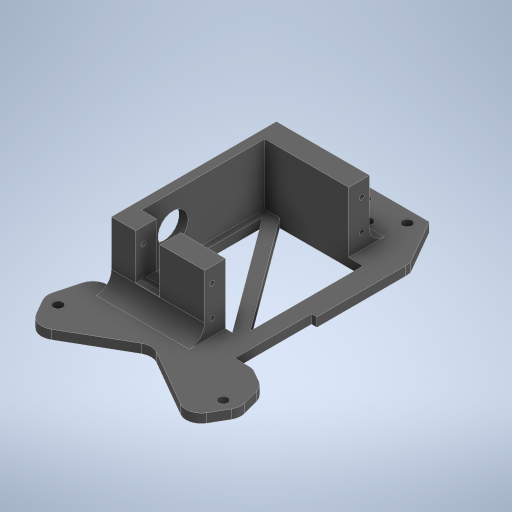
# Autodesk Inventor part: upper_arm_base
Saved by Autodesk Inventor 2024.1 (Build 281209000, 209)
## iProperties
Created: 2025-03-03
Part Number: upper_arm_base
Material: 一般
Document SubType Name: Modeling
Designer: hibik
Density: 1 g/cm^3
Appearance: 既定
Author: hibik
Autodesk Inventor part; units mm, degrees
ref_plane "XZ Plane" through (0, 0, 0) normal (0, 1, 0) x (-1, 0, 0)
ref_plane "XY Plane" through (0, 0, 0) normal (0, 0, 1) x (1, 0, 0)
ref_plane "作業平面1" through (7.8, 0, 0) normal (1, 0, 0) x (0, 1, 0)
sketch "スケッチ1" plane through (7.8, 0, 0) normal (1, 0, 0) x (0, 1, 0)
  line L0 (0, 27.3) -> (-20.1, 27.3)
  line L1 (-20.1, 27.3) -> (-20.1, 20.4)
  line L2 (-20.1, 20.4) -> (0, 20.4)
  line L3 (0, 20.4) -> (0, 27.3)
  line L4 (0, -20.4) -> (-20.1, -20.4)
  line L5 (-20.1, -20.4) -> (-20.1, -27.3)
  line L6 (-20.1, -27.3) -> (0, -27.3)
  line L7 (0, -27.3) -> (0, -20.4)
  line L8 (0, -38.22) -> (0, 38.22) projected
  line L9 (-24.12, 0) -> (4.02, 0) projected
  point P0 (0, 0)
  dimension "d1" = 40.8
  dimension "d3" = 20.1
  dimension "d13" = 6.9
  constraints: 16 end point, 4 parallel, 3 collinear, 2 horizontal, 2 perpendicular, 1 point on line, 1 other
  measures "d1" distance between parallel lines of L4 L2
  measures "d3" distance of L5.end L6.end
  measures "d13" distance of L2.end L0.start
extrude "押し出し1" add sketch "スケッチ1" against normal blind 27.8
sketch "スケッチ2" plane through (-20, 0, 0) normal (-1, 0, 0) x (0, 0, 1)
  line L0 (27.3, 0) -> (27.3, -20.1) projected
  line L1 (-27.3, -20.1) -> (-20.4, -20.1) projected
  line L2 (27.3, 0) -> (-27.3, 0)
  line L3 (-27.3, 0) -> (-27.3, -20.1)
  line L4 (-27.3, -20.1) -> (27.3, -20.1)
  line L5 (27.3, -20.1) -> (27.3, 0)
  point P0 (0, 0)
  constraints: 8 end point, 2 parallel, 1 horizontal, 1 perpendicular
extrude "押し出し2" add sketch "スケッチ2" along normal blind 3
sketch "スケッチ3" plane through (-23, 0, 0) normal (-1, 0, 0) x (0, 0, 1)
  circle A0 centre (9.9, -10.5) radius 5
  line L0 (27.3, 0) -> (-27.3, 0) projected
  line L1 (20.4, 0) -> (20.4, -20.1) projected
  point P0 (0, 0)
  dimension "d8" = 10
  dimension "d9" = 10.5
  dimension "d10" = 10.5
  constraints: 1 centre point
  measures "d8" diameter of A0
  measures "d9" distance from line of L0 A0.centre
  measures "d10" distance from line of L1 A0.centre
extrude "押し出し3" cut sketch "スケッチ3" against normal through all
sketch "スケッチ7" plane through (7.8, 0, 0) normal (1, 0, 0) x (0, 0, -1)
  arc A0 (-26.6208, -6.3) -> (-26.6208, -3.8) centre (-24.75, -5.05) ccw projected
  arc A1 (-26.6208, -16.3) -> (-26.6208, -13.8) centre (-24.75, -15.05) ccw projected
  arc A2 (26.6208, -3.8) -> (26.6208, -6.3) centre (24.75, -5.05) ccw projected
  arc A3 (26.6208, -13.8) -> (26.6208, -16.3) centre (24.75, -15.05) ccw projected
  circle A4 centre (-24.75, -5.05) radius 0.85
  circle A5 centre (-24.75, -15.05) radius 0.85
  circle A6 centre (24.75, -5.05) radius 0.85
  circle A7 centre (24.75, -15.05) radius 0.85
  point P0 (0, 0)
  dimension "d25" = 1.7
  constraints: 4 centre point, 3 coincident, 3 equal radius, 1 concentric
  measures "d25" diameter of A4
extrude "押し出し6" cut sketch "スケッチ7" against normal through all
sketch "スケッチ9" plane through (7.8, -20.1, -27.3) normal (0, -1, 0) x (1, 0, 0)
  line L0 (-32.5673, -16.6603) -> (18.1673, -16.6603)
  line L1 (18.1673, -16.6603) -> (55.6673, 48.2917)
  line L2 (55.6673, 48.2917) -> (30.3, 92.2291)
  line L3 (30.3, 92.2291) -> (-44.7, 92.2291)
  line L4 (-44.7, 92.2291) -> (-70.0673, 48.2917)
  line L5 (-70.0673, 48.2917) -> (-32.5673, -16.6603)
  line L6 (0, 0) -> (-30.8, 0) projected
  line L7 (11.8, 54.6) -> (-26.2, 54.6)
  line L8 (-26.2, 54.6) -> (-26.2, 0) construction
  line L9 (-26.2, 0) -> (11.8, 0)
  line L10 (11.8, 0) -> (11.8, 54.6)
  line L11 (0, 6.9) -> (0, 0) projected
  line L12 (0, 54.6) -> (-30.8, 54.6) projected
  line L13 (-142.2, 119.2291) -> (-7.2, -114.5977)
  line L14 (-7.2, -114.5977) -> (127.8, 119.2291)
  line L15 (-37.5673, -8) -> (-27.175, -2)
  line L16 (-27.175, -2) -> (-7.2, -2)
  line L17 (-142.2, 119.2291) -> (127.8, 119.2291)
  line L18 (-7.2, -2) -> (-7.2, -16.6603) construction
  line L19 (23.1673, -8) -> (12.775, -2)
  line L20 (12.775, -2) -> (-7.2, -2)
  line L21 (-26.0203, -2) -> (-17.5562, -16.6603)
  line L22 (11.6203, -2) -> (3.1562, -16.6603)
  line L23 (-57.3837, 70.2604) -> (36.9173, 15.8157) construction
  line L24 (42.9837, 70.2604) -> (-51.3173, 15.8157) construction
  line L25 (50.6673, 39.6314) -> (40.275, 45.6314)
  line L26 (40.275, 45.6314) -> (30.2875, 62.9303)
  line L27 (20.3, 80.2291) -> (30.2875, 62.9303)
  line L28 (20.3, 92.2291) -> (20.3, 80.2291)
  line L29 (20.8774, 79.2291) -> (37.8056, 79.2291)
  line L30 (39.6977, 46.6314) -> (48.1618, 61.2917)
  line L31 (-34.7, 92.2291) -> (-34.7, 80.2291)
  line L32 (-34.7, 80.2291) -> (-44.6875, 62.9303)
  line L33 (-54.675, 45.6314) -> (-44.6875, 62.9303)
  line L34 (-65.0673, 39.6314) -> (-54.675, 45.6314)
  line L35 (-54.0977, 46.6314) -> (-62.5618, 61.2917)
  line L36 (-35.2774, 79.2291) -> (-52.2056, 79.2291)
  line L37 (-54.0977, 46.6314) -> (-26.0203, -2) construction
  line L38 (11.6203, -2) -> (39.6977, 46.6314) construction
  line L39 (-35.2774, 79.2291) -> (20.8774, 79.2291) construction
  line L40 (18.5679, 79.2291) -> (38.543, 44.6314)
  line L41 (-32.9679, 79.2291) -> (-52.943, 44.6314)
  line L42 (-34.7, 80.2291) -> (-7.2, 64.352)
  line L43 (-7.2, 64.352) -> (20.3, 80.2291)
  line L44 (11.8, 29.1913) -> (40.275, 45.6314)
  line L45 (-54.675, 45.6314) -> (-30.8, 31.8472)
  line L46 (-30.8, 0) -> (-30.8, 54.6) projected
  line L47 (-26.0203, -2) -> (-27.175, 0)
  line L48 (11.6203, -2) -> (11.8, 0)
  point P0 (-7.8, 27.3)
  point P1 (-7.2, 92.2291)
  point P2 (-7.2, 0)
  point P3 (-7.2, 41.2868)
  point P4 (-32.9679, 79.2291)
  point P5 (-52.943, 44.6314)
  dimension "d29" = 38
  dimension "d30" = 26.2
  dimension "d34" = 270
  dimension "d35" = 75
  dimension "d37" = 27
  dimension "d38" = 27
  dimension "d40" = 10
  dimension "d41" = 12
  dimension "d42" = 27
  dimension "d43" = 1
  dimension "d44" = 1
  dimension "d45" = 2
  dimension "d48" = 360
  dimension "d50" = 2
  dimension "d51" = 2
  constraints: 90 end point, 17 point on line, 9 parallel, 7 midpoint, 7 perpendicular, 6 horizontal, 5 equal length, 2 symmetric about line, 1 coincident, 1 collinear, 1 vertical alignment, 46 other
  measures "d29" distance of L8.end L9.end
  measures "d30" distance between parallel lines of L8 L11
  measures "d34" distance of L14.end L13.start
  measures "d35" distance of L2.end L3.end
  measures "d37" distance between parallel lines of L13 L5
  measures "d38" distance between parallel lines of L14 L1
  measures "d40" distance from line of L0.start L15
  measures "d41" distance from line of L15.end L5
  measures "d42" distance between parallel lines of L17 L3
  measures "d43" distance from line of L15.end L21
  measures "d44" distance from line of L20.start L22
  measures "d45" distance between parallel lines of L6 L16
  measures "d50" distance between parallel lines of L27 L40
  measures "d51" distance between parallel lines of L32 L41
extrude "押し出し7" add sketch "スケッチ9" along normal blind 3 contours L21 L16 L20 L22 L0 | L47 L6 L9 L48 L20 L16 | L6 L46 L12 L7 L10 L9 | L41 L42 L43 L40 L44 L10 L7 L12 L46 L45
sketch "スケッチ12" plane through (7.8, -20.1, -27.3) normal (0, 1, 0) x (1, 0, 0)
  line L0 (0, -47.7) -> (0, -54.6) projected
  line L1 (0, -54.6) -> (10, -54.6)
  line L2 (10, -54.6) -> (10, -29.6)
  line L3 (10, -29.6) -> (0, -29.6)
  line L4 (0, -29.6) -> (0, -54.6)
  line L5 (11.8, 0) -> (11.8, -29.1913) projected
  line L6 (10, -54.6) -> (16, -54.6)
  line L7 (16, -54.6) -> (16, -29.1913)
  line L8 (16, -29.1913) -> (10, -29.1913)
  line L9 (10, -29.1913) -> (10, -54.6)
  line L10 (0, -54.6) -> (-30.8, -54.6) projected
  line L11 (-30.8, -54.6) -> (-47.1876, -54.6)
  line L12 (-32.9679, -79.2291) -> (-52.943, -44.6314) projected
  line L13 (-52.943, -44.6314) -> (-30.8, -31.8472) projected
  line L14 (-30.8, -54.6) -> (-30.8, 0) projected
  point P0 (-7.8, -27.3)
  dimension "d59" = 25
  dimension "d60" = 10
  dimension "d61" = 6
  constraints: 18 end point, 4 parallel, 3 horizontal, 2 perpendicular, 2 point on line
  measures "d59" distance of L1.end L2.end
  measures "d60" distance of L0.end L1.end
  measures "d61" distance of L1.end L6.end
extrude "押し出し9" cut sketch "スケッチ12" against normal through all contours L2 L9 L8 L7 L6 | L11 L12 L13 L14
sketch "スケッチ13" plane through (7.8, -20.1, -27.3) normal (0, 1, 0) x (1, 0, 0)
  circle A0 centre (-0.2, 12.6603) radius 1.6
  circle A1 centre (-14.2, 12.6603) radius 1.6
  line L0 (-17.5562, 16.6603) -> (3.1562, 16.6603) projected
  line L1 (-7.2, 16.6603) -> (-7.2, 5.6822)
  line L2 (-17.5562, 16.6603) -> (3.1562, 16.6603) projected
  circle A2 centre (-34.5038, -68.5689) radius 1.6
  circle A3 centre (-44.4789, -51.2917) radius 1.6
  line L3 (-32.9679, -79.2291) -> (-52.943, -44.6314) projected
  line L4 (-42.9555, -61.9303) -> (-35.2404, -57.476)
  line L5 (-7.2, -64.352) -> (-32.9679, -79.2291) projected
  line L6 (-7.2, -64.352) -> (-7.2, -38.8829)
  circle A4 centre (20.1038, -68.5689) radius 1.6
  circle A5 centre (30.0789, -51.2917) radius 1.6
  point P0 (-7.8, -27.3)
  dimension "d64" = 3.2
  dimension "d65" = 4
  dimension "d66" = 7
  dimension "d75" = 10
  dimension "d76" = 4
  constraints: 6 centre point, 6 end point, 4 symmetric about line, 3 equal radius, 2 midpoint, 2 perpendicular, 1 vertical, 2 other
  measures "d64" diameter of A0
  measures "d65" distance from line of L0 A0.centre
  measures "d66" distance from line of L1 A0.centre
  measures "d75" distance from line of L5 A2.centre
  measures "d76" distance from line of L3 A2.centre
extrude "押し出し10" cut sketch "スケッチ13" against normal through all
sketch "スケッチ14" plane through (7.8, -20.1, -27.3) normal (0, 1, 0) x (1, 0, 0)
  line L0 (4.8, -47.7) -> (-25.8, -47.7)
  line L1 (-25.8, -47.7) -> (-25.8, -6.9)
  line L2 (-25.8, -6.9) -> (4.8, -6.9)
  line L3 (4.8, -6.9) -> (4.8, -47.7)
  line L4 (0, -47.7) -> (-27.8, -47.7) projected
  line L5 (-27.8, -47.7) -> (-27.8, -6.9) projected
  line L6 (0, -6.9) -> (-27.8, -6.9) projected
  line L7 (-30.8, -31.8472) -> (-30.8, 0) projected
  line L8 (11.8, 0) -> (11.8, -29.1913) projected
  line L9 (3.1906, -48.8873) -> (6.4094, -46.5127)
  line L10 (6.4094, -46.5127) -> (-23.6906, -5.7127)
  line L11 (-23.6906, -5.7127) -> (-26.9094, -8.0873)
  line L12 (-26.9094, -8.0873) -> (3.1906, -48.8873)
  line L13 (16, -54.6) -> (10, -54.6) projected
  line L14 (16, -54.6) -> (28.5907, -61.8692)
  line L15 (38.543, -44.6314) -> (18.5679, -79.2291) projected
  circle A0 centre (-14.2, 12.6603) radius 1.6 projected
  circle A1 centre (-0.2, 12.6603) radius 1.6 projected
  line L16 (16, -31.6162) -> (16, -54.6) projected
  line L17 (16, -54.6) -> (10, -54.6) projected
  line L18 (10, -54.6) -> (10, -29.1913) projected
  line L19 (10, -29.1913) -> (11.8, -29.1913) projected
  line L20 (11.8, 0) -> (11.8, -29.1913) projected
  line L21 (11.6203, 2) -> (11.8, 0) projected
  line L22 (3.1562, 16.6603) -> (11.6203, 2) projected
  line L23 (-17.5562, 16.6603) -> (3.1562, 16.6603) projected
  line L24 (-27.175, 0) -> (-17.5562, 16.6603) projected
  line L25 (0, 0) -> (-27.175, 0) projected
  line L26 (0, -6.9) -> (0, 0) projected
  line L27 (0, -6.9) -> (-27.8, -6.9) projected
  line L28 (-27.8, -6.9) -> (-27.8, -47.7) projected
  line L29 (0, -47.7) -> (-27.8, -47.7) projected
  line L30 (0, -54.6) -> (0, -47.7) projected
  line L31 (0, -54.6) -> (-30.8, -54.6) projected
  line L32 (-32.9679, -79.2291) -> (-47.1876, -54.6) projected
  line L33 (-7.2, -64.352) -> (-32.9679, -79.2291) projected
  line L34 (18.5679, -79.2291) -> (-7.2, -64.352) projected
  line L35 (38.543, -44.6314) -> (18.5679, -79.2291) projected
  line L36 (16, -31.6162) -> (38.543, -44.6314) projected
  circle A2 centre (-31.6735, -71.7906) radius 2.8438
  circle A3 centre (-40.8912, -49.9054) radius 3.5315
  line L37 (-30.8, -54.6) -> (-47.1876, -54.6) projected
  point P0 (-7.8, -27.3)
  point P1 (-22.8, -6.9)
  point P2 (-25.3, -6.9)
  point P3 (-22.8146, -6.9)
  point P4 (4.8, -44.3311)
  point P5 (2.3146, -47.7)
  point P6 (-25.8, -9.5911)
  dimension "d69" = 5
  dimension "d70" = 7
  dimension "d71" = 4
  constraints: 18 end point, 4 parallel, 3 perpendicular, 2 centre point, 2 collinear, 2 midpoint, 2 point on line, 1 horizontal
  measures "d69" distance between parallel lines of L7 L1
  measures "d70" distance between parallel lines of L8 L3
  measures "d71" distance between parallel lines of L12 L10
extrude "押し出し11" cut sketch "スケッチ14" against normal through all contours L0 L1 L12 | L10 L2 L3 | L14 L16 L36 L15
fillet "フィレット2" radius 5 2 edges at (-7.6, -20.1, 27.3) (-5.7875, -20.1, -27.3)
sketch "スケッチ16" plane through (7.8, -20.1, -27.3) normal (0, 1, 0) x (1, 0, 0)
  line L0 (-39.4555, -67.9924) -> (-36.8933, -58.4303)
  line L1 (-36.8933, -58.4303) -> (-46.4555, -55.8681)
  line L2 (-32.9679, -79.2291) -> (-52.943, -44.6314) projected
  line L3 (28.5907, -61.8692) -> (18.5679, -79.2291) projected
  line L4 (25.0907, -67.9314) -> (22.5285, -58.3692)
  line L5 (28.5907, -61.8692) -> (16, -54.6) projected
  line L6 (-36.8933, -58.4303) -> (-42.9555, -61.9303)
  line L7 (-36.8933, -58.4303) -> (-35.867, -54.6)
  line L8 (-35.867, -54.6) -> (-47.1876, -54.6)
  line L9 (-46.4555, -55.8681) -> (-47.1876, -54.6)
  line L10 (-30.8, -54.6) -> (-47.1876, -54.6) projected
  point P0 (-7.8, -27.3)
  dimension "d78" = 7
  dimension "d79" = 7
  dimension "d80" = 7
  dimension "d81" = 7
  constraints: 14 end point, 4 point on line, 2 equal length, 2 perpendicular, 1 collinear, 1 horizontal, 1 midpoint
  measures "d78" distance from line of L0.start L6
  measures "d79" distance from line of L0.end L2
  measures "d80" distance from line of L4.end L3
  measures "d81" distance from line of L4.start L5
extrude "押し出し12" cut sketch "スケッチ16" against normal through all
sketch "スケッチ17" plane through (-23, 0, 27.3) normal (0, 0, 1) x (1, 0, 0)
  line L0 (30.8, 0) -> (0, 0) projected
  line L1 (8, 0) -> (16, 0)
  line L2 (16, 0) -> (16, -15)
  line L3 (16, -15) -> (8, -15)
  line L4 (8, -15) -> (8, 0)
  line L5 (3, -5.5) -> (3, -15.5) projected
  line L6 (3, -20.1) -> (3, 0) projected
  line L7 (3, 0) -> (3, -20.1) projected
  point P0 (23, 0)
  dimension "d84" = 15
  dimension "d89" = 5
  dimension "d90" = 13
  constraints: 8 end point, 2 parallel, 1 horizontal, 1 perpendicular, 1 point on line
  measures "d84" distance of L1.end L2.end
  measures "d89" distance between parallel lines of L4 L6
  measures "d90" distance between parallel lines of L6 L2
extrude "押し出し13" cut sketch "スケッチ17" against normal up to surface (6.9 mm away)
sketch "スケッチ18" plane through (7.8, -20.1, -27.3) normal (0, 1, 0) x (1, 0, 0)
  circle A0 centre (-7.2, 6.6603) radius 1.6
  circle A1 centre (-0.2, 12.6603) radius 1.6 projected
  circle A2 centre (-14.2, 12.6603) radius 1.6 projected
  point P0 (-7.8, -27.3)
  dimension "d91" = 3.2
  dimension "d92" = 7
  dimension "d93" = 7
  dimension "d94" = 6
  constraints: 1 centre point
  measures "d91" diameter of A0
  measures "d92" horizontal distance of A0.centre A1.centre
  measures "d93" horizontal distance of A2.centre A0.centre
  measures "d94" vertical distance of A2.centre A0.centre
extrude "押し出し14" cut sketch "スケッチ18" against normal through all contours A0
fillet "フィレット3" radius 5 8 edges at (-25.1679, -21.6, 51.9291) (26.3679, -21.6, 51.9291) (32.8907, -21.6, 40.6314) (-31.6555, -21.6, 40.6924) (30.3285, -21.6, 31.0692) (23.8, -21.6, 27.3) (0.6, -21.6, 37.052) (-28.067, -21.6, 27.3)
equation "\"d37\" = d42"
equation "\"d38\" = d42"
equation "\"d44\" = d43"
equation "\"d50\" = d45"
equation "\"d51\" = d50"
equation "\"d76\" = d65"
equation "\"d80\" = d79"
equation "\"d81\" = d78"
equation "\"d92\" = d93"
